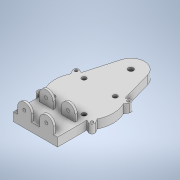
# Autodesk Inventor part: GripperBase
Saved by Autodesk Inventor 2020 (Build 240168000, 168)
## iProperties
Created: 2019-11-04
Part Number: GripperBase
Material: Generic
Document SubType Name: Modeling
Designer: kaspe
Density: 1 g/cm^3
Appearance: Default
Author: kaspe
Autodesk Inventor part; units mm, degrees
ref_plane "YZ Plane" through (0, 0, 0) normal (1, 0, 0) x (0, 1, 0)
sketch "Sketch1" plane through (0, 0, 0) normal (0, 1, 0) x (-1, 0, 0)
  circle A0 centre (0, 0) radius 31.65
  circle A1 centre (0, 0) radius 33.15
  dimension "d0" = 63.3
  dimension "d1" = 66.3
  constraints: 2 centre point, 2 coincident
  measures "d0" diameter of A0
  measures "d1" diameter of A1
sketch "Sketch1 outline for Extrusion1" plane through (0, 0, 0) normal (0, 1, 0) x (-1, 0, 0)
  circle A0 centre (0, 0) radius 33.15
extrude "Extrusion1" add sketch "Sketch1 outline for Extrusion1" along normal blind 9.8
sketch "Sketch2" plane through (0, 0, 0) normal (0, -1, 0) x (1, 0, 0)
  circle A0 centre (0, 0) radius 31.65
  dimension "d4" = 63.3
  constraints: 1 centre point, 1 coincident
  measures "d4" diameter of A0
sketch "Sketch2 outline for Extrusion2" plane through (0, 0, 0) normal (0, -1, 0) x (1, 0, 0)
  circle A0 centre (0, 0) radius 31.65
extrude "Extrusion2" cut sketch "Sketch2 outline for Extrusion2" against normal blind 6.5
sketch "Sketch3" plane through (0, 9.8, 0) normal (0, 1, 0) x (1, 0, 0)
  circle A0 centre (0, 0) radius 25
  line L0 (0, 0) -> (17.67767, 17.67767)
  line L1 (0, 0) -> (25, 0) construction
  line L2 (0, 0) -> (-17.67767, 17.67767)
  line L3 (0, 0) -> (-17.67767, -17.67767)
  line L4 (0, 0) -> (17.67767, -17.67767)
  circle A1 centre (-17.67767, 17.67767) radius 2.55
  circle A2 centre (17.67767, 17.67767) radius 2.55
  circle A3 centre (17.67767, -17.67767) radius 2.55
  circle A4 centre (-17.67767, -17.67767) radius 2.55
  circle A5 centre (0, 25) radius 3.05
  dimension "d7" = 50
  dimension "d8" = 45
  dimension "d9" = 5.1
  dimension "d10" = 5.1
  dimension "d11" = 5.1
  dimension "d12" = 5.1
  dimension "d13" = 6.1
  constraints: 10 end point, 6 centre point, 6 point on circle, 4 coincident, 1 equal length, 1 horizontal, 1 perpendicular, 1 point on line
  measures "d7" diameter of A0
  measures "d8" angle of L1 L0
  measures "d9" diameter of A1
  measures "d10" diameter of A2
  measures "d11" diameter of A3
  measures "d12" diameter of A4
  measures "d13" diameter of A5
sketch "Sketch3 outline for Extrusion3" plane through (0, 9.8, 0) normal (0, 1, 0) x (1, 0, 0)
  circle A0 centre (17.67767, -17.67767) radius 2.55
  circle A1 centre (17.67767, 17.67767) radius 2.55
  circle A2 centre (0, 25) radius 3.05
  circle A3 centre (-17.67767, 17.67767) radius 2.55
  circle A4 centre (-17.67767, -17.67767) radius 2.55
extrude "Extrusion3" cut sketch "Sketch3 outline for Extrusion3" against normal blind 6.5
sketch "Sketch4" plane through (0, 9.8, 0) normal (0, 1, 0) x (1, 0, 0)
  circle A0 centre (0, 0) radius 33.15 projected
  line L0 (0, 33.15) -> (0, -33.15)
  constraints: 2 end point, 2 point on circle, 1 vertical
ref_plane "Work Plane1" through (0, 9.8, 33.15) normal (0, 0, 1) x (1, 0, 0)
ref_plane "Work Plane2" through (0, 9.8, -33.15) normal (0, 0, -1) x (-1, 0, 0)
sketch "Sketch5" plane through (0, 9.8, -33.15) normal (0, 0, -1) x (-1, 0, 0)
  line L0 (33.15, 0) -> (-33.15, 0) projected
  line L1 (0, 0) -> (25, 0)
  line L2 (0, 0) -> (-25, 0)
  line L3 (33.15, -9.8) -> (-33.15, -9.8) projected
  line L4 (-25, 0) -> (25, 0)
  line L5 (25, 0) -> (25, -9.8)
  line L6 (25, -9.8) -> (-25, -9.8)
  line L7 (-25, -9.8) -> (-25, 0)
  point P0 (0, -9.8)
  dimension "d16" = 25
  dimension "d17" = 25
  constraints: 12 end point, 3 point on line, 2 parallel, 1 horizontal, 1 midpoint, 1 perpendicular
  measures "d16" distance of L1.start L1.end
  measures "d17" distance of L1.start L2.end
sketch "Sketch5 outline for Extrusion4" plane through (0, 9.8, -33.15) normal (0, 0, -1) x (-1, 0, 0)
  line L0 (-25, 0) -> (-25, -9.8)
  line L1 (25, 0) -> (-25, 0)
  line L2 (25, -9.8) -> (25, 0)
  line L3 (-25, -9.8) -> (25, -9.8)
extrude "Extrusion4" add sketch "Sketch5 outline for Extrusion4" against normal blind 11.75
sketch "Sketch6" plane through (0, 9.8, 33.15) normal (0, 0, 1) x (1, 0, 0)
  line L0 (-25, 0) -> (25, 0) projected
  line L1 (0, 0) -> (-25, 0)
  line L2 (-25, 0) -> (-25, -9.8) projected
  line L3 (25, -9.8) -> (25, 0) projected
  line L4 (-25, 0) -> (25, 0)
  line L5 (25, 0) -> (25, -9.8)
  line L6 (25, -9.8) -> (-25, -9.8)
  line L7 (-25, -9.8) -> (-25, 0)
  point P0 (0, -9.8)
  dimension "d20" = 25
  dimension "d21" = 50
  constraints: 10 end point, 2 parallel, 1 collinear, 1 horizontal, 1 midpoint, 1 perpendicular
  measures "d20" distance of L1.start L0.start
  measures "d21" distance of L3.start L6.end
sketch "Sketch6 outline for Extrusion5" plane through (0, 9.8, 33.15) normal (0, 0, 1) x (1, 0, 0)
  line L0 (-25, -9.8) -> (25, -9.8)
  line L1 (-25, 0) -> (-25, -9.8)
  line L2 (25, 0) -> (-25, 0)
  line L3 (25, -9.8) -> (25, 0)
extrude "Extrusion5" add sketch "Sketch6 outline for Extrusion5" against normal blind 12.25
sketch "Sketch8" plane through (0, 9.8, 33.15) normal (0, 0, 1) x (1, 0, 0)
  line L0 (-25, -9.8) -> (25, -9.8) projected
  line L1 (25, 0) -> (25, -9.8) projected
  line L2 (-25, -9.8) -> (25, -9.8)
  line L3 (25, -9.8) -> (25, 0)
  line L4 (25, 0) -> (-25, 0)
  line L5 (-25, 0) -> (-25, -9.8)
  point P0 (0, -9.8)
  constraints: 8 end point, 2 parallel, 1 horizontal, 1 perpendicular
sketch "Sketch8 outline for Extrusion6" plane through (0, 9.8, 33.15) normal (0, 0, 1) x (1, 0, 0)
  line L0 (-25, 0) -> (-25, -9.8)
  line L1 (25, 0) -> (-25, 0)
  line L2 (25, -9.8) -> (25, 0)
  line L3 (-25, -9.8) -> (25, -9.8)
extrude "Extrusion6" add sketch "Sketch8 outline for Extrusion6" along normal blind 22
sketch "Sketch9" plane through (0, 9.8, 0) normal (0, 1, 0) x (1, 0, 0)
  line L0 (-25, -55.15) -> (-25, -21.769761)
  line L1 (25, -21.769761) -> (25, -55.15)
  line L2 (-25, -55.15) -> (25, -55.15)
  line L3 (25, -55.15) -> (25, -52.65)
  line L4 (25, -52.65) -> (-25, -52.65)
  line L5 (-25, -52.65) -> (-25, -55.15)
  point P0 (0, 0)
  dimension "d26" = 2.5
  constraints: 8 end point, 2 parallel, 1 horizontal, 1 perpendicular, 1 point on line
  measures "d26" distance of L3.end L2.end
sketch "Sketch9 outline for Extrusion7" plane through (0, 9.8, 0) normal (0, 1, 0) x (1, 0, 0)
  line L0 (-25, -55.15) -> (25, -55.15)
  line L1 (-25, -52.65) -> (-25, -55.15)
  line L2 (25, -52.65) -> (-25, -52.65)
  line L3 (25, -55.15) -> (25, -52.65)
extrude "Extrusion7" add sketch "Sketch9 outline for Extrusion7" along normal blind 19
sketch "Sketch11" plane through (0, 9.8, 0) normal (0, 1, 0) x (1, 0, 0)
  line L0 (25, -21.769761) -> (25, -52.65)
  line L1 (-25, -52.65) -> (-25, -21.769761)
  line L2 (25, -52.65) -> (-25, -52.65)
  line L3 (-25, -52.65) -> (-25, -30.55)
  line L4 (-25, -30.55) -> (25, -30.55)
  line L5 (25, -30.55) -> (25, -52.65)
  line L6 (25, -30.55) -> (-25, -30.55)
  line L7 (-25, -30.55) -> (-25, -28.05)
  line L8 (-25, -28.05) -> (25, -28.05)
  line L9 (25, -28.05) -> (25, -30.55)
  point P0 (0, 0)
  dimension "d39" = 22.1
  dimension "d40" = 2.5
  constraints: 16 end point, 4 parallel, 2 horizontal, 2 perpendicular, 2 point on line
  measures "d39" distance of L2.end L3.end
  measures "d40" distance of L6.end L7.end
sketch "Sketch11 outline for Extrusion9" plane through (0, 9.8, 0) normal (0, 1, 0) x (1, 0, 0)
  line L0 (25, -28.05) -> (-25, -28.05)
  line L1 (25, -30.55) -> (25, -28.05)
  line L2 (-25, -30.55) -> (25, -30.55)
  line L3 (-25, -28.05) -> (-25, -30.55)
extrude "Extrusion9" add sketch "Sketch11 outline for Extrusion9" along normal blind 19
sketch "Sketch10" plane through (0, 9.8, 55.15) normal (0, 0, 1) x (1, 0, 0)
  line L0 (-25, 0) -> (25, 0) projected
  line L1 (25, -9.8) -> (25, 19) projected
  line L2 (-25, 0) -> (25, 0)
  line L3 (25, 0) -> (25, 7.8)
  line L4 (25, 7.8) -> (-25, 7.8)
  line L5 (-25, 7.8) -> (-25, 0)
  line L6 (0, 0) -> (12.5, 0)
  line L7 (0, 0) -> (-12.5, 0)
  circle A0 centre (-12.5, 7.8) radius 1.75
  circle A1 centre (12.5, 7.8) radius 1.75
  point P0 (0, -9.8)
  dimension "d29" = 7.8
  dimension "d30" = 12.5
  dimension "d31" = 12.5
  dimension "d32" = 3.5
  dimension "d33" = 3.5
  constraints: 12 end point, 5 point on line, 2 centre point, 2 parallel, 1 horizontal, 1 midpoint, 1 perpendicular
  measures "d29" distance of L3.end L2.end
  measures "d30" distance of L6.start L6.end
  measures "d31" distance of L6.start L7.end
  measures "d32" diameter of A0
  measures "d33" diameter of A1
sketch "Sketch10 outline for Extrusion8" plane through (0, 9.8, 55.15) normal (0, 0, 1) x (1, 0, 0)
  circle A0 centre (12.5, 7.8) radius 1.75
  circle A1 centre (-12.5, 7.8) radius 1.75
extrude "Extrusion8" cut sketch "Sketch10 outline for Extrusion8" against normal blind 32.5
chamfer "Chamfer2" distance 10 angle 45 4 edges at (-25, 28.8, 29.3) (25, 28.8, 29.3) (25, 28.8, 53.9) (-25, 28.8, 53.9)
sketch "Sketch12" plane through (0, 9.8, -33.15) normal (0, 0, -1) x (-1, 0, 0)
  point P0 (0, -9.8)
sketch "Sketch13" plane through (0, 9.8, -33.15) normal (0, 0, -1) x (-1, 0, 0)
  line L0 (-25, 0) -> (-33.15, 0) projected
  line L1 (25, -9.8) -> (-25, -9.8) projected
  line L2 (-25, 0) -> (25, 0)
  line L3 (25, 0) -> (25, -9.8)
  line L4 (25, -9.8) -> (-25, -9.8)
  line L5 (-25, -9.8) -> (-25, 0)
  point P0 (0, -9.8)
  constraints: 8 end point, 2 parallel, 1 horizontal, 1 perpendicular
sketch "Sketch13 outline for Extrusion10" plane through (0, 9.8, -33.15) normal (0, 0, -1) x (-1, 0, 0)
  line L0 (25, -9.8) -> (25, 0)
  line L1 (-25, -9.8) -> (25, -9.8)
  line L2 (-25, 0) -> (-25, -9.8)
  line L3 (25, 0) -> (-25, 0)
extrude "Extrusion10" add sketch "Sketch13 outline for Extrusion10" along normal blind 35.5
sketch "Sketch14" plane through (0, 9.8, 0) normal (0, 1, 0) x (1, 0, 0)
  line L0 (25, 68.65) -> (-25, 68.65) projected
  line L1 (0, 68.65) -> (0, 53.15)
  circle A0 centre (0, 53.15) radius 3
  point P0 (0, 0)
  dimension "d48" = 15.5
  dimension "d49" = 6
  constraints: 2 end point, 1 centre point, 1 coincident, 1 midpoint, 1 vertical
  measures "d48" distance of L1.start L1.end
  measures "d49" diameter of A0
sketch "Sketch14 outline for Extrusion11" plane through (0, 9.8, 0) normal (0, 1, 0) x (1, 0, 0)
  circle A0 centre (0, 53.15) radius 3
extrude "Extrusion11" cut sketch "Sketch14 outline for Extrusion11" against normal blind 32.5
sketch "Sketch15" plane through (0, 9.8, 0) normal (0, 1, 0) x (1, 0, 0)
  circle A0 centre (0, 53.15) radius 3
  circle A1 centre (0, 53.15) radius 15.5
  line L0 (25, 21.769761) -> (25, 68.65)
  line L1 (25, 21.769761) -> (14.913097, 57.37487)
  line L2 (-25, 68.65) -> (-25, 21.769761)
  line L3 (-25, 21.769761) -> (-14.913097, 57.37487)
  arc A2 (25, -21.769761) -> (25, 21.769761) centre (0, 0) ccw
  arc A3 (-25, 21.769761) -> (-25, -21.769761) centre (0, 0) ccw
  arc A4 (25, 21.769761) -> (-25, 21.769761) centre (0, 0) ccw
  line L4 (25, 68.65) -> (-25, 68.65)
  line L5 (-25, 68.65) -> (-25, 21.769761)
  line L6 (-25, 21.769761) -> (25, 21.769761)
  line L7 (25, 21.769761) -> (25, 68.65)
  point P0 (0, 68.65)
  dimension "d52" = 31
  constraints: 12 end point, 4 point on circle, 2 centre point, 2 parallel, 2 tangent, 1 coincident, 1 horizontal, 1 perpendicular
  measures "d52" diameter of A1
sketch "Sketch15 outline for Extrusion12" plane through (0, 9.8, 0) normal (0, 1, 0) x (1, 0, 0)
  line L0 (25, 68.65) -> (0, 68.65)
  line L1 (25, 21.769761) -> (25, 68.65)
  line L2 (14.913097, 57.37487) -> (25, 21.769761)
  arc A0 (0, 68.65) -> (14.913097, 57.37487) centre (0, 53.15) cw
  line L3 (0, 68.65) -> (-25, 68.65)
  arc A1 (-14.913097, 57.37487) -> (0, 68.65) centre (0, 53.15) cw
  line L4 (-25, 21.769761) -> (-14.913097, 57.37487)
  line L5 (-25, 68.65) -> (-25, 21.769761)
extrude "Extrusion12" cut sketch "Sketch15 outline for Extrusion12" against normal blind 32.5
sketch "Sketch16" plane through (0, 9.8, 0) normal (0, 1, 0) x (1, 0, 0)
  arc A0 (25, -21.769761) -> (25, 21.769761) centre (0, 0) ccw
  line L0 (0, 0) -> (33.15, 0) construction
  line L1 (0, 0) -> (33.15, 0) construction
  arc A1 (-25, 21.769761) -> (-25, -21.769761) centre (0, 0) ccw
  circle A2 centre (29.658128, -20.66748) radius 1.65
  circle A3 centre (29.612346, 20.734788) radius 1.65
  circle A4 centre (-29.732977, 20.730735) radius 1.65
  circle A5 centre (-29.612346, -20.734788) radius 1.65
  arc A6 (-32.18532, -19.192126) -> (-28.262212, -23.413806) centre (-29.612346, -20.734788) ccw
  arc A7 (-28.424016, 23.430109) -> (-32.341269, 19.24857) centre (-29.732977, 20.730735) ccw
  line L2 (-29.732977, 20.730735) -> (-25.86811, 20.730735)
  line L3 (29.650842, -14.82397) -> (32.230672, -19.124102)
  line L4 (29.618676, 14.888134) -> (32.188973, 19.198236)
  line L5 (-29.732977, 14.658533) -> (-32.341269, 19.24857)
  line L6 (-29.612346, -14.900719) -> (-32.18532, -19.192126)
  line L7 (25, 21.769761) -> (28.262212, 23.413806)
  line L8 (-14.913097, 57.37487) -> (-25, 21.769761)
  line L9 (-25, 21.769761) -> (-28.424016, 23.430109)
  line L10 (-25, -21.769761) -> (-28.262212, -23.413806)
  line L11 (25, -21.769761) -> (25, -28.05)
  line L12 (25, -21.769761) -> (28.366796, -23.375332)
  arc A8 (32.188973, 19.198236) -> (28.262212, 23.413806) centre (29.612346, 20.734788) ccw
  arc A9 (27.24024, -18.89158) -> (26.65813, -20.671221) centre (29.658128, -20.66748) ccw
  arc A10 (28.366796, -23.375332) -> (32.230672, -19.124102) centre (29.658128, -20.66748) ccw
  point P0 (25.86811, 20.730735)
  point P1 (25.914954, -20.672148)
  point P2 (27.15489, 19.014059)
  point P3 (26.612348, 20.73154)
  point P4 (27.15489, -19.014059)
  dimension "d58" = 3.3
  dimension "d62" = 3.3
  dimension "d63" = 3.3
  constraints: 22 end point, 19 point on circle, 9 centre point, 8 tangent, 4 coincident, 2 horizontal, 1 point on line
  measures "d58" diameter of A2
  measures "d62" diameter of A3
  measures "d63" diameter of A4
sketch "Sketch16 outline for Extrusion13" plane through (0, 9.8, 0) normal (0, 1, 0) x (1, 0, 0)
  arc A0 (28.366796, -23.375332) -> (32.230672, -19.124102) centre (29.658128, -20.66748) ccw
  line L0 (25, -21.769761) -> (28.366796, -23.375332)
  line L1 (32.230672, -19.124102) -> (29.650842, -14.82397)
  arc A1 (29.650842, -14.82397) -> (25, -21.769761) centre (0, 0) cw
  circle A2 centre (29.658128, -20.66748) radius 1.65
  arc A3 (-32.18532, -19.192126) -> (-28.262212, -23.413806) centre (-29.612346, -20.734788) ccw
  line L2 (-29.612346, -14.900719) -> (-32.18532, -19.192126)
  line L3 (-28.262212, -23.413806) -> (-25, -21.769761)
  arc A4 (-25, -21.769761) -> (-29.612346, -14.900719) centre (0, 0) cw
  circle A5 centre (-29.612346, -20.734788) radius 1.65
  arc A6 (-29.732977, 14.658533) -> (-25, 21.769761) centre (0, 0) cw
  line L4 (-32.341269, 19.24857) -> (-29.732977, 14.658533)
  line L5 (-25, 21.769761) -> (-28.424016, 23.430109)
  arc A7 (-28.424016, 23.430109) -> (-32.341269, 19.24857) centre (-29.732977, 20.730735) ccw
  circle A8 centre (-29.732977, 20.730735) radius 1.65
  arc A9 (32.188973, 19.198236) -> (28.262212, 23.413806) centre (29.612346, 20.734788) ccw
  line L6 (29.618676, 14.888134) -> (32.188973, 19.198236)
  line L7 (28.262212, 23.413806) -> (25, 21.769761)
  arc A10 (25, 21.769761) -> (29.618676, 14.888134) centre (0, 0) cw
  circle A11 centre (29.612346, 20.734788) radius 1.65
extrude "Extrusion13" add sketch "Sketch16 outline for Extrusion13" against normal up to surface (9.8 mm away)
sketch "Sketch17" plane through (0, 6.5, 0) normal (0, -1, 0) x (1, 0, 0)
  circle A0 centre (0, 0) radius 31.65
  constraints: 1 centre point, 1 coincident
sketch "Sketch17 outline for Extrusion14" plane through (0, 6.5, 0) normal (0, -1, 0) x (1, 0, 0)
  circle A0 centre (0, 0) radius 31.65
extrude "Extrusion14" cut sketch "Sketch17 outline for Extrusion14" along normal blind 10
sketch "Sketch18" plane through (0, 0, 0) normal (0, -1, 0) x (1, 0, 0)
  circle A0 centre (0, -53.15) radius 3
  line L0 (0, -53.15) -> (0, -58.15)
  line L1 (0, -53.15) -> (0, -48.15)
  line L2 (0, -53.15) -> (-5.75, -53.15)
  line L3 (0, -53.15) -> (5.75, -53.15)
  line L4 (-5.75, -53.15) -> (-2.875, -58.15)
  line L5 (-2.875, -58.15) -> (2.875, -58.15)
  line L6 (2.875, -58.15) -> (5.75, -53.15)
  line L7 (5.75, -53.15) -> (2.875, -48.190625)
  line L8 (2.875, -48.190625) -> (-3, -48.190625)
  line L9 (-3, -48.190625) -> (-5.75, -53.15)
  circle A1 centre (0, -53.15) radius 3
  point P0 (0, 0)
  dimension "d70" = 5
  dimension "d72" = 5.75
  constraints: 20 end point, 3 horizontal, 2 vertical, 1 centre point, 1 coincident, 1 perpendicular
  measures "d70" distance of L0.start L1.end
  measures "d72" distance of L0.start L3.end
sketch "Sketch18 outline for Extrusion15" plane through (0, 0, 0) normal (0, -1, 0) x (1, 0, 0)
  line L0 (-2.875, -58.15) -> (2.875, -58.15)
  line L1 (-5.75, -53.15) -> (-2.875, -58.15)
  line L2 (2.875, -58.15) -> (5.75, -53.15)
  line L3 (-3, -48.190625) -> (-5.75, -53.15)
  line L4 (5.75, -53.15) -> (2.875, -48.190625)
  line L5 (2.875, -48.190625) -> (-3, -48.190625)
  circle A0 centre (0, -53.15) radius 3
extrude "Extrusion15" cut sketch "Sketch18 outline for Extrusion15" against normal blind 5
sketch "Sketch19" plane through (25, 9.8, 28.05) normal (0, 0, -1) x (-1, 0, 0)
  circle A0 centre (12.5, 7.8) radius 1.75
  circle A1 centre (12.5, 7.8) radius 7.8
  line L0 (39.913097, 0) -> (10.086903, 0)
  circle A2 centre (37.5, 7.8) radius 1.75
  circle A3 centre (37.5, 7.8) radius 7.8
  line L1 (29.7, 7.8) -> (29.7, 0)
  line L2 (45.3, 7.8) -> (45.3, 0)
  line L3 (0, 0) -> (50, 0)
  line L4 (20.3, 7.8) -> (20.3, 0)
  line L5 (4.7, 7.8) -> (4.7, 0)
  line L6 (0, 0) -> (53.091017, 0)
  line L7 (53.091017, 0) -> (53.091017, 22.153705)
  line L8 (53.091017, 22.153705) -> (0, 22.153705)
  line L9 (0, 22.153705) -> (0, 0)
  point P0 (25, -9.8)
  constraints: 16 end point, 4 parallel, 4 point on circle, 4 point on line, 3 perpendicular, 3 tangent, 2 centre point, 2 coincident, 1 horizontal
sketch "Sketch19 outline for Extrusion16" plane through (25, 9.8, 28.05) normal (0, 0, -1) x (-1, 0, 0)
  line L0 (0, 22.153705) -> (0, 0)
  line L1 (53.091017, 22.153705) -> (0, 22.153705)
  line L2 (53.091017, 0) -> (53.091017, 22.153705)
  line L3 (50, 0) -> (53.091017, 0)
  line L4 (45.3, 0) -> (50, 0)
  line L5 (45.3, 7.8) -> (45.3, 0)
  arc A0 (29.7, 7.8) -> (45.3, 7.8) centre (37.5, 7.8) cw
  line L6 (29.7, 0) -> (29.7, 7.8)
  line L7 (20.3, 0) -> (29.7, 0)
  line L8 (20.3, 7.8) -> (20.3, 0)
  arc A1 (4.7, 7.8) -> (20.3, 7.8) centre (12.5, 7.8) cw
  line L9 (4.7, 0) -> (4.7, 7.8)
  line L10 (0, 0) -> (4.7, 0)
extrude "Extrusion16" cut sketch "Sketch19 outline for Extrusion16" against normal blind 52
body "Solid1"
